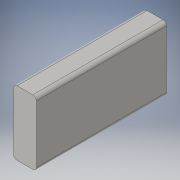
# Autodesk Inventor part: BATTARY
Saved by Autodesk Inventor 2016 (Build 200138000, 138)
## iProperties
Created: 2016-10-04
Part Number: BATTARY
Material: Generic
Document SubType Name: Modeling
Designer: brandn
Density: 1 g/cm^3
Appearance: Default
Author: brandn
Autodesk Inventor part; units mm, degrees
ref_plane "YZ Plane" through (0, 0, 0) normal (1, 0, 0) x (0, 1, 0)
ref_plane "XZ Plane" through (0, 0, 0) normal (0, 1, 0) x (-1, 0, 0)
ref_plane "XY Plane" through (0, 0, 0) normal (0, 0, 1) x (1, 0, 0)
sketch "Sketch1" plane through (0, 0, 0) normal (1, 0, 0) x (0, 1, 0)
  line L0 (10.9447, 32.8342) -> (-23.4723, 32.8342)
  line L1 (-23.4723, 32.8342) -> (-23.4723, -36.4824)
  line L2 (-23.4723, -36.4824) -> (10.9447, -36.4824)
  line L3 (10.9447, -36.4824) -> (10.9447, 32.8342)
  point P0 (0, 0)
  dimension "d0" = 69.3166
  dimension "d1" = 34.417
  constraints: 8 end point, 2 parallel, 1 horizontal, 1 perpendicular
  measures "d0" distance of L2.end L0.start
  measures "d1" distance of L0.start L0.end
extrude "Extrusion1" add sketch "Sketch1" along normal blind 12.2428
fillet "Fillet1" radius 1.905 4 edges at (12.2428, 10.9447, -1.8241) (0, 10.9447, -1.8241) (12.2428, -23.4723, -1.8241) (0, -23.4723, -1.8241)
body "Solid1"
